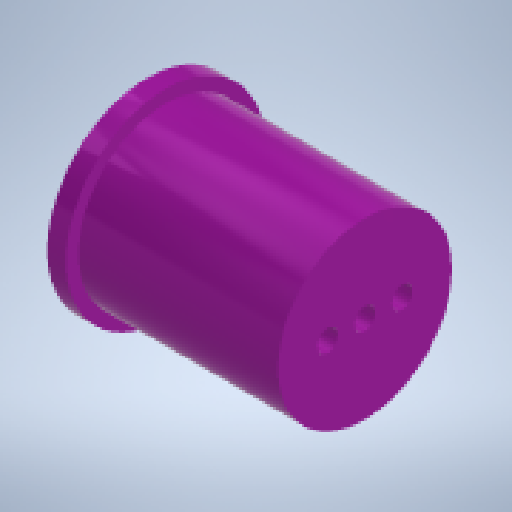
# Autodesk Inventor part: 028
Saved by Autodesk Inventor 2023 (Build 270158000, 158)
## iProperties
Created: 2022-04-04
Part Number: 028
Material: PC/ABS Plastic
Document SubType Name: Modeling
Designer: Vinicius Miguel
Density: 0.357273 g/cm^3
Appearance: Smooth - Purple
Mass: 6.10297 g
Surface Area: 114.249 cm^2
Volume: 17.0821 cm^3
Author: Vinicius Miguel
Autodesk Inventor part; units mm, degrees
ref_plane "YZ Plane" through (0, 0, 0) normal (1, 0, 0) x (0, 1, 0)
ref_plane "XZ Plane" through (0, 0, 0) normal (0, 1, 0) x (-1, 0, 0)
ref_plane "XY Plane" through (0, 0, 0) normal (0, 0, 1) x (1, 0, 0)
sketch "Sketch1" plane through (0, 0, 0) normal (0, 1, 0) x (-1, 0, 0)
  line L0 (0, 0) -> (35, 0)
  line L1 (35, 0) -> (35, -16)
  line L2 (35, -16) -> (32, -16)
  line L3 (32, -16) -> (32, -14)
  line L4 (32, -14) -> (0, -14)
  line L5 (0, -14) -> (0, 0)
  line L6 (35, 0) -> (45, 0)
  line L7 (45, 0) -> (45, -11)
  line L8 (45, -11) -> (35, -11)
  line L9 (5, 0) -> (5, -11)
  line L10 (5, -11) -> (45, -11)
  line L11 (27, -14) -> (27, -12.8)
  line L12 (27, -12.8) -> (29, -12.8)
  line L13 (29, -12.8) -> (29, -14)
  point P0 (35, -11)
  point P1 (32, -15)
  point P2 (27, -11)
  point P3 (29, -11)
  dimension "d0" = 28
  dimension "d1" = 32
  dimension "d2" = 3
  dimension "d3" = 35
  dimension "d5" = 10
  dimension "d6" = 5
  dimension "d7" = 3
  dimension "d18" = 2
  dimension "d20" = 22
  dimension "d21" = 3
  dimension "d24" = 1.2
  constraints: 28 end point, 11 perpendicular, 5 point on line, 2 horizontal, 1 midpoint, 1 vertical
  measures "d0" diameter of L4 L0
  measures "d1" diameter of L2 L0
  measures "d2" distance of L1.end L2.end
  measures "d3" distance of L0.start L0.end
  measures "d5" distance of L7.end L8.end
  measures "d6" distance between parallel lines of L5 L9
  measures "d7" distance between parallel lines of L4 L10
  measures "d18" distance of L11.end L12.end
  measures "d20" diameter of L8 L0
  measures "d21" horizontal distance of L13.end point (32, -15)
  measures "d24" distance of L12.end L13.end
revolve "Revolution1" add sketch "Sketch1" angle 360 about axis through (0, 0, 0) along (-1, 0, 0) contours L0 L9 L10 L1 L2 L3 L4 L13 L12 L11 L5
sketch "Sketch2" plane through (0, 0, 0) normal (1, 0, 0) x (0, 0, -1)
  point P0 (0, 0)
  point P1 (0, 0)
  point P2 (6, 0)
  point P3 (-6, 0)
  dimension "d22" = 6
  dimension "d23" = 6
  constraints: 2 horizontal alignment, 1 coincident
  measures "d22" distance of point (0, 0) point (-6, 0)
  measures "d23" distance of point (6, 0) point (0, 0)
hole "Hole1" at (0, 0, 0) at (0, 0, -6) at (0, 0, 6) direction (-1, 0, 0) diameter 3.4 end through all clearance for "Countersunk Flat Head Screw ISO 2009/7046" size "M3" standard "ISO"
equation "\"d23\" = d22"
body "Solid1"
